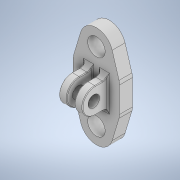
# Autodesk Inventor part: itemMount
Saved by Autodesk Inventor 2021.3 (Build 253353010, 353A)
## iProperties
Created: 2021-08-11
Part Number: itemMount
Material: Generisch
Document SubType Name: Modeling
Designer: Markus
Density: 1 g/cm^3
Appearance: Vorgabe
Author: Markus
Autodesk Inventor part; units mm, degrees
ref_plane "YZ Plane" through (0, 0, 0) normal (1, 0, 0) x (0, 1, 0)
ref_plane "XZ Plane" through (0, 0, 0) normal (0, 1, 0) x (-1, 0, 0)
ref_plane "XY Plane" through (0, 0, 0) normal (0, 0, 1) x (1, 0, 0)
sketch "Skizze1" plane through (0, 0, 0) normal (0, 0, 1) x (1, 0, 0)
  line L0 (-4.535, 4.95) -> (-1.535, 4.95)
  line L1 (-1.535, 4.95) -> (-1.535, -4.95)
  line L2 (-1.535, -4.95) -> (-4.535, -4.95)
  line L3 (-4.535, -4.95) -> (-4.535, 4.95)
  line L4 (1.535, 4.95) -> (4.535, 4.95)
  line L5 (4.535, 4.95) -> (4.535, -4.95)
  line L6 (4.535, -4.95) -> (1.535, -4.95)
  line L7 (1.535, -4.95) -> (1.535, 4.95)
  line L8 (0, 4.95) -> (0, -4.95) construction
  point P0 (0, 0)
  point P1 (-1.535, 0)
  dimension "d0" = 3
  dimension "d1" = 9.9
  dimension "d2" = 3.07
  constraints: 18 end point, 4 parallel, 3 horizontal alignment, 2 horizontal, 2 midpoint, 2 perpendicular, 1 vertical, 4 other
  measures "d0" distance of L0.start L0.end
  measures "d1" distance of L2.end L0.start
  measures "d2" distance between parallel lines of L7 L1
extrude "Extrusion1" add sketch "Skizze1" along normal blind 10
sketch "Skizze2" plane through (4.535, -4.95, 0) normal (1, 0, 0) x (0, 0, -1)
  line L0 (0, 9.9) -> (-10, 9.9) projected
  arc A0 (-5.05, 9.9) -> (-5.05, 0) centre (-5.05, 4.95) ccw
  line L1 (-10, 9.9) -> (-10, 0) projected
  line L2 (0, 0) -> (-10, 0) projected
  line L3 (-5.05, 9.9) -> (0, 9.9)
  line L4 (0, 0) -> (0, 9.9) projected
  line L5 (0, 9.9) -> (0, 0)
  line L6 (0, 0) -> (-5, 0)
  line L7 (0, 0) -> (-10, 0) projected
  circle A1 centre (-5.55, 4.95) radius 2.25
  point P0 (0, 4.95)
  point P1 (-10, 4.95)
  dimension "d5" = 4.5
  dimension "d7" = 0.5
  constraints: 6 end point, 3 tangent, 2 centre point, 2 point on circle, 2 point on line, 1 horizontal alignment, 1 midpoint, 1 perpendicular
  measures "d5" diameter of A1
  measures "d7" distance of A1.centre A0.centre
extrude "Extrusion2" cut sketch "Skizze2" against normal up to surface (9.07 mm away) contours A0 L1 L0 | A0 L2 L1 | A1
sketch "Skizze3" plane through (0, 0, 0) normal (0, 0, -1) x (-1, 0, 0)
  line L0 (9, 4.95) -> (9, -4.95)
  line L1 (-9, -4.95) -> (-9, 4.95)
  line L2 (1.535, 4.95) -> (4.535, 4.95) projected
  line L3 (4.535, 4.95) -> (4.535, -4.95) projected
  arc A0 (6.1266, 15.2007) -> (-6.1266, 15.2007) centre (0, 13.35) ccw
  circle A1 centre (0, 13.35) radius 3.4
  line L4 (0, 9.95) -> (0, -9.95) construction
  line L5 (-9, 0) -> (9, 0) construction
  arc A2 (-8.7864, 6.3959) -> (-9, 4.95) centre (-4, 4.95) ccw
  arc A3 (9, 4.95) -> (8.7864, 6.3959) centre (4, 4.95) ccw
  line L6 (6.1266, 15.2007) -> (8.7864, 6.3959)
  line L7 (-6.1266, 15.2007) -> (-8.7864, 6.3959)
  arc A4 (-6.1266, -15.2007) -> (6.1266, -15.2007) centre (0, -13.35) ccw
  circle A5 centre (0, -13.35) radius 3.4
  arc A6 (-9, -4.95) -> (-8.7864, -6.3959) centre (-4, -4.95) ccw
  arc A7 (8.7864, -6.3959) -> (9, -4.95) centre (4, -4.95) ccw
  line L8 (6.1266, -15.2007) -> (8.7864, -6.3959)
  line L9 (-6.1266, -15.2007) -> (-8.7864, -6.3959)
  line L10 (-1.535, 4.95) -> (-4.535, 4.95) projected
  point P0 (0, 0)
  point P1 (0, -9.95)
  point P2 (-3.035, 4.95)
  dimension "d13" = 6.8
  dimension "d12" = 3
  dimension "d15" = 18
  dimension "d19" = 5
  dimension "d21" = 5
  constraints: 16 end point, 14 point on circle, 12 symmetric about line, 7 centre point, 6 tangent, 3 coincident, 3 midpoint, 3 vertical alignment, 2 horizontal alignment, 1 horizontal, 1 parallel, 1 point on line, 1 vertical, 9 other
  measures "d15" distance between parallel lines of L0 L1
  measures "d19" radius of A2
  measures "d21" distance from line of L2 point (0, 9.95)
extrude "Extrusion3" add sketch "Skizze3" along normal blind 5
fillet "Rundung1" radius 0.5 4 edges at (4.535, 0, 0) (1.535, 0, 0) (-4.535, 0, 0) (-1.535, 0, 0)
fillet "Rundung2" radius 2 12 edges at (4.785, 4.95, 0) (3.035, 4.95, 0) (1.285, 4.95, 0) (-4.785, 4.95, 0) (-3.035, 4.95, 0) (-1.285, 4.95, 0) (-4.785, -4.95, 0) (-3.035, -4.95, 0) (-1.285, -4.95, 0) (4.785, -4.95, 0) (3.035, -4.95, 0) (1.285, -4.95, 0)
fillet "Rundung3" radius 0.25 28 edges at (4.535, 0, 10) (4.535, -4.95, 3.525) (4.535, -5.1271, 1.1771) (4.7041, -6.2535, 0.1252) (4.535, 5.1271, 1.1771) (4.7041, 6.2535, 0.1252) (4.535, 4.95, 3.525) (-1.535, 0, 10) (-1.535, -4.95, 3.525) (-1.535, -5.1271, 1.1771) (-1.3659, -6.2535, 0.1252) (-1.535, 5.1271, 1.1771) (-1.3659, 6.2535, 0.1252) (-1.535, 4.95, 3.525) (1.535, 0, 10) (1.535, -4.95, 3.525) (1.535, -5.1271, 1.1771) (1.3659, -6.2535, 0.1252) (1.535, 5.1271, 1.1771) (1.3659, 6.2535, 0.1252) (1.535, 4.95, 3.525) (-4.535, 0, 10) (-4.535, -4.95, 3.525) (-4.535, -5.1271, 1.1771) (-4.7041, -6.2535, 0.1252) (-4.535, 5.1271, 1.1771) (-4.7041, 6.2535, 0.1252) (-4.535, 4.95, 3.525)
